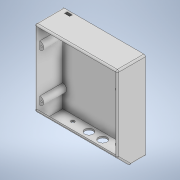
# Autodesk Inventor part: mávač_krabička
Saved by Autodesk Inventor 2022 (Build 260153000, 153)
## iProperties
Created: 2022-06-10
Part Number: mávač_krabička
Material: Generic
Document SubType Name: Modeling
Designer: Ruslana Zubareva
Density: 1 g/cm^3
Appearance: Default
Author: Ruslana Zubareva
Autodesk Inventor part; units mm, degrees
ref_plane "YZ Plane" through (0, 0, 0) normal (1, 0, 0) x (0, 1, 0)
sketch "Sketch1" plane through (0, 0, 0) normal (0, 0, 1) x (1, 0, 0)
  line L0 (0, 0) -> (150, 0)
  line L1 (150, 0) -> (150, -160)
  line L2 (150, -160) -> (0, -160)
  line L3 (0, -160) -> (0, 0)
  dimension "d0" = 150
  dimension "d1" = 160
  constraints: 8 end point, 2 parallel, 1 horizontal, 1 perpendicular
  measures "d0" distance of L1.end L2.end
  measures "d1" distance of L0.end L1.end
extrude "Extrusion1" add sketch "Sketch1" along normal blind 50
chamfer "Chamfer1" distance 25 angle 45 1 edges at (75, -160, 50)
shell "Shell1" thickness 3 outward yes removed faces 1 at (50, -45, 50)
fillet "Fillet1" radius 3 7 edges at (153, 3, 23.5) (-3, 3, 23.5) (-3, -151.1213, 38.1213) (153, -151.1213, 38.1213) (-3, -163, 11.6213) (153, -163, 11.6213) (75, -163, 26.2426)
fillet "Fillet2" radius 3 8 edges at (-2.1213, -138, 50) (75, -139.2426, 50) (152.1213, -138, 50) (153, -67.5, 50) (152.1213, 2.1213, 50) (75, 3, 50) (-2.1213, 2.1213, 50) (-3, -67.5, 50)
sketch "Sketch3" plane through (0, -162.1213, 27.1213) normal (0, -0.7071068, 0.7071068) x (1, 0, 0)
  line L0 (0, 35.3553) -> (0, 130.8148) projected
  line L1 (0, -17.6777) -> (0, 0) projected
  circle A0 centre (75, 16.6122) radius 7.5
  line L2 (0, 0) -> (0, 31.1127) projected
  line L3 (67.5, 16.6122) -> (27.5, 16.6122)
  circle A1 centre (27.5, 16.6122) radius 6
  line L4 (82.5, 16.6122) -> (122.5, 16.6122)
  circle A2 centre (122.5, 16.6122) radius 6
  point P0 (0, 95.4594)
  dimension "d12" = 15
  dimension "d13" = 75
  dimension "d18" = 40
  dimension "d19" = 12
  dimension "d20" = 40
  dimension "d21" = 12
  constraints: 4 end point, 3 centre point, 2 coincident, 2 point on circle, 2 point on line, 1 horizontal
  measures "d12" diameter of A0
  measures "d13" distance from line of L2 A0.centre
  measures "d18" distance of L3.start L3.end
  measures "d19" diameter of A1
  measures "d20" distance of L4.start L4.end
  measures "d21" diameter of A2
extrude "Extrusion2" cut sketch "Sketch3" against normal blind 10 contours A0
extrude "Extrusion3" cut sketch "Sketch3" against normal blind 10 contours A1 | A2
sketch "Sketch4" plane through (0, -163, -3) normal (0, -1, 0) x (1, 0, 0)
  line L0 (0, 28) -> (150, 28) projected
  line L1 (0, 28) -> (150, 28) projected
  line L2 (75, 28) -> (75, 3.5926)
  line L3 (150, 28) -> (150, 0) projected
  line L4 (150, 14) -> (120, 14)
  line L5 (0, 3) -> (0, 28) projected
  line L6 (0, 14) -> (30, 14)
  circle A0 centre (30, 14) radius 3.25
  circle A1 centre (120, 14) radius 3.25
  dimension "d24" = 30
  dimension "d26" = 30
  dimension "d27" = 6.5
  dimension "d28" = 6.5
  constraints: 6 end point, 2 centre point, 2 coincident, 2 horizontal, 2 midpoint, 1 point on line, 1 vertical
  measures "d24" distance of L4.start L4.end
  measures "d26" distance of L6.start L6.end
  measures "d27" diameter of A0
  measures "d28" diameter of A1
extrude "Extrusion4" cut sketch "Sketch4" against normal blind 10
sketch "Sketch5" plane through (0, -163, -3) normal (0, -1, 0) x (1, 0, 0)
  line L0 (0, 28) -> (150, 28) projected
  line L1 (75, 28) -> (75, 3)
  line L2 (150, 3) -> (0, 3) projected
  line L3 (62, 15.5) -> (88, 15.5)
  circle A0 centre (88, 15.5) radius 8
  circle A1 centre (62, 15.5) radius 8
  dimension "d31" = 26
  dimension "d32" = 16
  dimension "d33" = 16
  constraints: 4 end point, 2 centre point, 2 coincident, 2 midpoint, 1 horizontal
  measures "d31" distance of L3.start L3.end
  measures "d32" diameter of A0
  measures "d33" diameter of A1
extrude "Extrusion5" cut sketch "Sketch5" against normal blind 10
sketch "Sketch6" plane through (0, 3, -3) normal (0, 1, 0) x (1, 0, 0)
  line L0 (150, -3) -> (0, -3) projected
  line L1 (8.7404, -3.5) -> (18.7404, -3.5)
  line L2 (18.7404, -3.5) -> (18.7404, -8.5)
  line L3 (18.7404, -8.5) -> (8.7404, -8.5)
  line L4 (8.7404, -8.5) -> (8.7404, -3.5)
  dimension "d36" = 10
  dimension "d37" = 5
  dimension "d49" = 0.5
  constraints: 8 end point, 2 parallel, 1 horizontal, 1 perpendicular
  measures "d36" distance of L2.end L3.end
  measures "d37" distance of L1.end L2.end
  measures "d49" distance between parallel lines of L0 L1
extrude "Extrusion6" cut sketch "Sketch6" against normal blind 10
sketch "Sketch10" plane through (0, 0, 0) normal (0, -1, 0) x (1, 0, 0)
  line L0 (0, 0) -> (0, 50) projected
  line L1 (3.7404, 12.4098) -> (43.7404, 12.4098)
  line L2 (43.7404, 12.4098) -> (43.7404, 0)
  line L3 (43.7404, 0) -> (3.7404, 0)
  line L4 (3.7404, 0) -> (3.7404, 12.4098)
  line L5 (8.7404, 5.5) -> (8.7404, 0.5) projected
  constraints: 8 end point, 2 parallel, 1 horizontal, 1 perpendicular
extrude "Extrusion8" cut sketch "Sketch10" against normal blind 2
sketch "Sketch11" plane through (0, -160, 0) normal (0, 0, 1) x (1, 0, 0)
  line L0 (0, 160) -> (0, 0) projected
  circle A0 centre (0, 125) radius 7.5
  line L1 (150, 163) -> (0, 163) projected
  circle A1 centre (3.5, 125) radius 1.5
  point P0 (0, 132.5)
  point P1 (0, 117.5)
  dimension "d52" = 15
  dimension "d53" = 38
  dimension "d54" = 3
  dimension "d55" = 3.5
  dimension "d56" = 38
  constraints: 2 centre point, 1 point on line
  measures "d52" diameter of A0
  measures "d53" distance from line of L1 A0.centre
  measures "d54" diameter of A1
  measures "d55" distance of A0.centre A1.centre
  measures "d56" distance from line of A1.centre L1
extrude "Extrusion9" add sketch "Sketch11" along normal blind 43 contours A0 L0 picked at (0.6667, 125)
sketch "Sketch12" plane through (3.5, -35, 0) normal (0, 0, 1) x (1, 0, 0)
  point P0 (-3.5, 35)
ref_plane "Work Plane2" through (75, -160, -3) normal (-1, 0, 0) x (0, 0, 1)
mirror "Mirror1" about plane through (75, -160, -3) normal (-1, 0, 0) of "Extrusion9"
ref_plane "Work Plane3" through (0, -80, -3) normal (0, 1, 0) x (1, 0, 0)
mirror "Mirror2" about plane through (0, -80, -3) normal (0, 1, 0) of "Extrusion9", "Mirror1"
body "Solid1"
